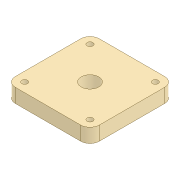
# Autodesk Inventor part: corpo_2_menor
Saved by Autodesk Inventor 2020 (Build 240168000, 168)
## iProperties
Created: 2022-07-20
Part Number: corpo_2_menor
Material: Genérico
Document SubType Name: Modeling
Designer: gabri
Density: 1 g/cm^3
Appearance: Bege
Author: gabri
Autodesk Inventor part; units mm, degrees
ref_plane "YZ Plane" through (0, 0, 0) normal (1, 0, 0) x (0, 1, 0)
ref_plane "XZ Plane" through (0, 0, 0) normal (0, 1, 0) x (-1, 0, 0)
ref_plane "XY Plane" through (0, 0, 0) normal (0, 0, 1) x (1, 0, 0)
sketch "Esboço1" plane through (0, 0, 0) normal (0, 1, 0) x (-1, 0, 0)
  circle A0 centre (0, 0) radius 7.55
  line L0 (0, 0) -> (36, 0)
  line L1 (36, 0) -> (36, -28)
  line L2 (28, -36) -> (0, -36)
  line L3 (0, -36) -> (0, 0)
  arc A1 (28, -36) -> (36, -28) centre (28, -28) ccw
  circle A2 centre (28, -28) radius 2.5
  point P0 (36, -36)
  point P1 (7.55, 0)
  point P2 (0, -7.55)
  dimension "d0" = 15.1
  dimension "d1" = 36
  dimension "d2" = 36
  dimension "d3" = 8
  dimension "d4" = 5
  dimension "d7" = 8
  dimension "d8" = 8
  constraints: 8 end point, 3 centre point, 2 coincident, 2 parallel, 2 point on circle, 2 point on line, 2 tangent, 1 horizontal, 1 perpendicular
  measures "d0" diameter of A0
  measures "d1" distance of point (36, -36) L2.end
  measures "d2" distance of L0.end point (36, -36)
  measures "d3" radius of A1
  measures "d4" diameter of A2
  measures "d7" distance of L1.end A1.centre
  measures "d8" distance from line of L2 A1.centre
extrude "Extrusão1" add sketch "Esboço1" along normal blind 12 contours L0 L1 A1 L2 L3 A0
mirror "Espelhamento1" about plane through (0, 0, -7.55) normal (1, 0, 0) of "Extrusão1"
mirror "Espelhamento2" about plane through (-36, 0, 0) normal (0, 0, 1) of "Extrusão1", "Espelhamento1"
